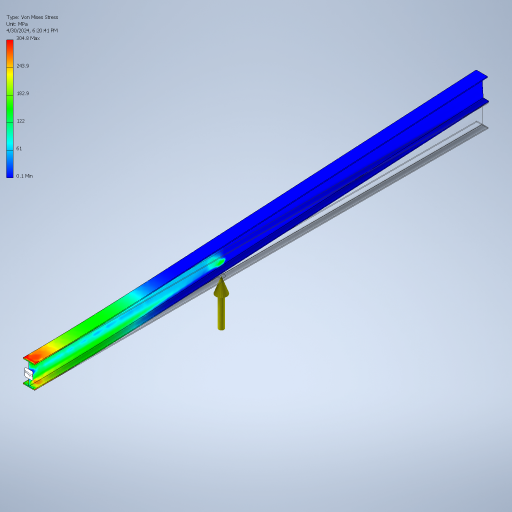
# Autodesk Inventor part: Part2
Saved by Autodesk Inventor 2024 (Build 280153000, 153)
## iProperties
Created: 2024-04-24
Part Number: Part2
Material: Aluminum 2014-T6
Document SubType Name: Modeling
Designer: AcerLaptopOwner
Mass: 21058.9 g
Surface Area: 31877.9 cm^2
Volume: 7549.97 cm^3
Density: 2.78927 g/cm^3
Appearance: Satin
Author: AcerLaptopOwner
Autodesk Inventor part; units mm, degrees
ref_plane "YZ Plane" through (0, 0, 0) normal (1, 0, 0) x (0, 1, 0)
ref_plane "XZ Plane" through (0, 0, 0) normal (0, 1, 0) x (-1, 0, 0)
ref_plane "XY Plane" through (0, 0, 0) normal (0, 0, 1) x (1, 0, 0)
sketch "Sketch1" plane through (0, 0, 0) normal (0, 1, 0) x (-1, 0, 0)
  point P0 (0, 0)
sketch "Sketch2" plane through (0, 0, 0) normal (0, 0, 1) x (1, 0, 0)
  line L0 (-50, 200) -> (50, 200)
  line L1 (50, 200) -> (50, 0)
  line L2 (50, 0) -> (-50, 0)
  line L3 (-50, 0) -> (-50, 200)
  line L4 (-50, 192.411) -> (-1, 192.411)
  line L5 (-1, 192.411) -> (-1, 7.589)
  line L6 (-1, 7.589) -> (-50, 7.589)
  line L7 (-50, 7.589) -> (-50, 192.411)
  line L8 (50, 192.411) -> (1, 192.411)
  line L9 (1, 192.411) -> (1, 7.589)
  line L10 (1, 7.589) -> (50, 7.589)
  line L11 (50, 7.589) -> (50, 192.411)
  point P0 (0, 0)
  point P1 (0, 0)
  dimension "d0" = 100
  dimension "d1" = 2
  dimension "d2" = 7.589
  dimension "d3" = 7.589
  dimension "d4" = 200
  constraints: 24 end point, 6 parallel, 4 point on line, 3 horizontal, 3 perpendicular, 1 coincident, 1 collinear, 1 midpoint
  measures "d0" distance of L0.start L0.end
  measures "d1" distance between parallel lines of L9 L5
  measures "d2" distance between parallel lines of L4 L0
  measures "d3" distance between parallel lines of L2 L6
  measures "d4" distance of L0.end L1.end
extrude "Extrusion1" add sketch "Sketch2" along normal blind 4000 contours L0 L1 L8 L9 L10 L2 L3 L6 L5 L4
sketch "Sketch3" plane through (-50, 0, 0) normal (0, -1, 0) x (1, 0, 0)
  line L0 (51, 0) -> (51, 4000) projected
  line L1 (0, 0) -> (0, 4000) projected
  line L2 (100, 0) -> (100, 4000) projected
  line L3 (0, 0) -> (0, 4000) projected
  line L4 (0, 2302.4) -> (100, 2302.4)
  line L5 (0, 0) -> (100, 0) projected
  circle A0 centre (50, 2302.4) radius 25
  point P0 (50, 0)
  point P1 (50, 0)
  dimension "d8" = 50
  dimension "d12" = 1697.6
  constraints: 2 end point, 2 midpoint, 2 point on line, 1 centre point, 1 parallel
  measures "d8" diameter of A0
  measures "d12" distance of L0.end A0.centre
extrude "Extrusion2" add sketch "Sketch3" along normal blind 0.1 contours A0 L4 L0 | L0 L4 A0 | L4 A0 L0 | L0 A0 L4
equation "\"d3\" = d2"
body "Solid1"
